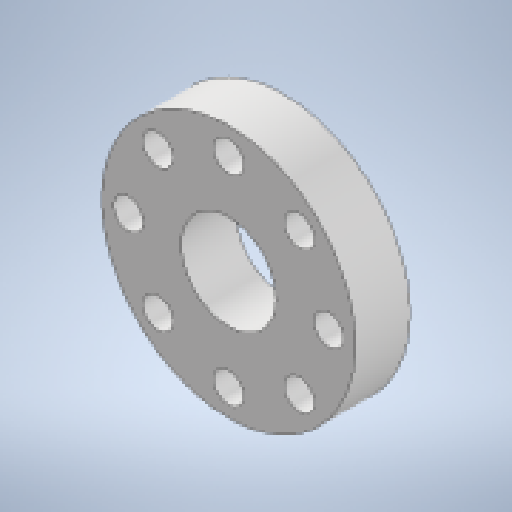
# Autodesk Inventor part: 부품71
Saved by Autodesk Inventor 2024 (Build 280153000, 153)
## iProperties
Created: 2024-09-08
Part Number: 부품71
Material: 일반
Document SubType Name: Modeling
Designer: Eungang
Density: 1 g/cm^3
Appearance: 기본값
Author: Eungang
Autodesk Inventor part; units mm, degrees
ref_plane "YZ Plane" through (0, 0, 0) normal (1, 0, 0) x (0, 1, 0)
ref_plane "XZ Plane" through (0, 0, 0) normal (0, 1, 0) x (-1, 0, 0)
ref_plane "XY Plane" through (0, 0, 0) normal (0, 0, 1) x (1, 0, 0)
sketch "스케치1" plane through (0, 0, 0) normal (0, 0, 1) x (1, 0, 0)
  circle A0 centre (0, 0) radius 13.9 projected
  circle A1 centre (0, 0) radius 5.2
  circle A2 centre (-7.7782, -7.7782) radius 1.65
  circle A3 centre (0, -11) radius 1.65
  circle A4 centre (7.7782, -7.7782) radius 1.65
  circle A5 centre (11, 0) radius 1.65
  circle A6 centre (7.7782, 7.7782) radius 1.65
  circle A7 centre (0, 11) radius 1.65
  circle A8 centre (-7.7782, 7.7782) radius 1.65
  circle A9 centre (-11, 0) radius 1.65
  point P0 (0, 0)
  dimension "d4" = 360
  constraints: 9 centre point, 17 other
extrude "돌출1" add sketch "스케치1" along normal blind 12
